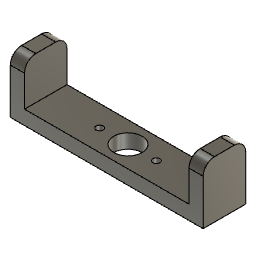
rubik_holder v10 (Autodesk Fusion 360 design; units mm, degrees)
Autodesk Fusion 360 part; units mm, degrees
sketch "Sketch1" plane through (0, 0, 0) normal (0, 0, 1) x (1, 0, 0)
  line L0 (34, -7.5) -> (-34, -7.5)
  line L1 (-34, -7.5) -> (-34, 7.5)
  line L2 (-34, 7.5) -> (34, 7.5)
  line L3 (34, 7.5) -> (34, -7.5)
  line L4 (34, -7.5) -> (-34, 7.5) construction
  line L5 (-34, -7.5) -> (34, 7.5) construction
  circle A0 centre (0, 0) radius 5
  line L6 (0, 0) -> (10, 0) construction
  circle A1 centre (10, 0) radius 1.25
  line L7 (0, 2.5) -> (0, 20)
  circle A2 centre (-10, 0) radius 1.25
  dimension "d18" = 68
  dimension "d19" = 15
  dimension "d20" = 10
  dimension "d22" = 10
  dimension "d23" = 2.5
  constraint horizontal L0
  constraint perpendicular L0 L1
  constraint parallel L0 L2
  constraint parallel L1 L3
  constraint coincident L4 A0.centre
  constraint coincident L5 A0.centre
  constraint coincident A0.centre L6.start
  constraint horizontal L6
  constraint coincident L6.end A1.centre
  constraint symmetric A1 L7 A2
  measures "d18" distance of L1.end L2.end
  measures "d19" distance of L0.start L2.end
  measures "d20" diameter of A0
  measures "d22" distance of A0.centre L6.end
  measures "d23" diameter of A1
extrude "Extrude1" add sketch "Sketch1" along normal blind 5
sketch "Sketch2" plane through (0, 0, 5) normal (0, 0, 1) x (-1, 0, 0)
  line L0 (0, -2.5) -> (0, -20)
  circle A0 centre (-10, 0) radius 1.25
  circle A1 centre (10, 0) radius 1.25
  circle A2 centre (0, 0) radius 5
  line L1 (-34, -7.5) -> (34, -7.5)
  line L2 (34, -7.5) -> (34, 7.5)
  line L3 (34, 7.5) -> (-34, 7.5)
  line L4 (-34, 7.5) -> (-34, -7.5)
  line L5 (34, -7.5) -> (29, -7.5)
  line L6 (29, -7.5) -> (29, 7.5)
  line L7 (29, 7.5) -> (34, 7.5)
  line L8 (34, 7.5) -> (34, -7.5)
  line L9 (-34, -7.5) -> (-29, -7.5)
  line L10 (-29, -7.5) -> (-29, 7.5)
  line L11 (-29, 7.5) -> (-34, 7.5)
  line L12 (-34, 7.5) -> (-34, -7.5)
  dimension "d24" = 5
  dimension "d25" = 5
  constraint perpendicular L5 L6
  constraint parallel L5 L7
  constraint parallel L6 L8
  constraint coincident L1 L5.end
  constraint perpendicular L2 L5
  constraint coincident L1.end L2.start
  constraint perpendicular L9 L10
  constraint parallel L9 L11
  constraint parallel L10 L12
  constraint coincident L1 L9.end
  constraint perpendicular L4 L9
  constraint coincident L1.start L4.end
  measures "d24" distance of L1.end L5.end
  measures "d25" distance of L1.start L9.end
extrude "Extrude2" add sketch "Sketch2" along normal blind 15 contours L1 L3 L4 L9 L10 L11 L12 | L1 L2 L3 L5 L6 L7 L8
fillet "Fillet2" radius 4 4 edges at (-31.5, -7.5, 20) (-31.5, 7.5, 20) (31.5, -7.5, 20) (31.5, 7.5, 20)
